Autodesk Inventor part; units mm, degrees
(part 2 of 2)
extrude "Extrusion24" cut sketch "Sketch28" against normal blind 1 contours L33 L34 L10 L12 | L12 L10 S18 L36 L29 L30 L31 L32 L33 | L12 L35 S16 S17 S18 L10 | L10 L34 L35 L12 | S2 S3 S4 S5 L13 L14 S6 S7 S8 S9 L10 | L10 S9 S10 S11 S12 S13 L15 L16 S14 S15 S0 S1 S2 | L26 L27 L28 L17 L18 L19 L20 L10 | L10 L20 L21 L22 L23 L24 L25 L26 | S25 S26 S27 S28 L40 L41 S29 S30 S31 S32 L10 | L10 S32 S33 S34 S35 S36 L42 L43 S37 S38 S23 S24 S25 bodies 3
chamfer "Chamfer2" distance 0.5 angle 45 69 edges at (3.5434, 22.1781, 13.5) (1.331, 22.8406, 13.5) (-2.8323, 22.4212, 13.5) (-6.3513, 18.4524, 13.5) (-6.3391, 11.8155, 13.5) (-2.814, 7.9075, 13.5) (1.3371, 7.5246, 13.5) (3.6102, 8.26, 13.5) (4.5462, 9.8949, 13.5) (3.7622, 10.527, 13.5) (4.4733, 11.0861, 13.5) (3.7075, 19.8625, 13.5) (1.4526, 21.0476, 13.5) (-1.9145, 20.8532, 13.5) (-4.4003, 17.7778, 13.5) (-4.3821, 12.5144, 13.5) (-1.8902, 9.5181, 13.5) (1.5012, 9.354, 13.5) (4.4672, 19.279, 13.5) (4.5462, 20.4824, 13.5) (5.8225, 21.9168, 13.5) (8.7277, 22.6826, 13.5) (6.7767, 21.151, 13.5) (7.731, 15.1826, 13.5) (9.7245, 15.1826, 13.5) (10.6787, 21.151, 13.5) (11.6329, 21.9168, 13.5) (8.7277, 7.6826, 13.5) (11.6329, 8.4484, 13.5) (10.6787, 9.2142, 13.5) (6.7767, 9.2142, 13.5) (5.8225, 8.4484, 13.5) (14.1005, 15.1826, 13.5) (16.0332, 22.6826, 13.5) (20.1236, 22.5428, 13.5) (23.0288, 20.5857, 13.5) (22.6459, 15.8572, 13.5) (16.9692, 15.3163, 13.5) (19.3942, 15.4682, 13.5) (16.094, 18.1364, 13.5) (19.4672, 20.841, 13.5) (17.0847, 20.9565, 13.5) (21.175, 19.6133, 13.5) (21.1994, 17.091, 13.5) (17.2366, 13.651, 13.5) (20.7496, 10.6668, 13.5) (16.094, 10.6668, 13.5) (15.0972, 7.6826, 13.5) (23.0409, 10.9464, 13.5) (24.4145, 7.6826, 13.5) (26.5417, 11.8155, 13.5) (26.5296, 18.4524, 13.5) (28.4988, 12.5144, 13.5) (28.4806, 17.7778, 13.5) (30.0669, 7.9075, 13.5) (34.218, 7.5246, 13.5) (30.9907, 9.5181, 13.5) (34.3821, 9.354, 13.5) (30.0486, 22.4212, 13.5) (34.2119, 22.8406, 13.5) (30.9664, 20.8532, 13.5) (34.3335, 21.0476, 13.5) (36.5883, 19.8625, 13.5) (37.4271, 20.4824, 13.5) (36.4242, 22.1781, 13.5) (37.4271, 9.8949, 13.5) (36.643, 10.527, 13.5) (36.4911, 8.26, 13.5) (37.3541, 11.0861, 13.5)
sketch "Sketch29" plane through (20, -26.8311, -2) normal (0.5, -0.8660254, 0) x (0.8660254, 0.5, 0)
  line L0 (33.3708, 0) -> (0, 0) projected
  line L1 (0, 7.25) -> (0, 0) projected
  line L2 (0, 7.25) -> (12.2679, 7.25) projected
  arc A0 (12.2679, 7.25) -> (16, 6.25) centre (14, 6.25) ccw projected
  arc A1 (16, 6.25) -> (15.7321, 7.25) centre (14, 6.25) ccw projected
  line L3 (15.7321, 7.25) -> (16.2679, 7.25) projected
  arc A2 (16.2679, 7.25) -> (16, 6.25) centre (18, 6.25) ccw projected
  line L4 (33.3708, 7.25) -> (33.3708, 0) projected
  line L5 (19.7321, 7.25) -> (33.3708, 7.25) projected
  arc A3 (16, 6.25) -> (19.7321, 7.25) centre (18, 6.25) ccw projected
  line L6 (0, 12.5) -> (33.3708, 12.5) projected
  line L7 (33.3708, 7.25) -> (33.3708, 12.5) projected
  line L8 (33.3708, 7.25) -> (19.7321, 7.25) projected
  arc A4 (19.7321, 7.25) -> (16.2679, 7.25) centre (18, 6.25) ccw projected
  line L9 (16.2679, 7.25) -> (15.7321, 7.25) projected
  arc A5 (15.7321, 7.25) -> (12.2679, 7.25) centre (14, 6.25) ccw projected
  line L10 (12.2679, 7.25) -> (0, 7.25) projected
  line L11 (0, 7.25) -> (0, 12.5) projected
  line L12 (16.2679, 5.25) -> (15.7321, 5.25) projected
  arc A6 (17.3708, 6.25) -> (17.6388, 5.25) centre (19.3708, 6.25) ccw projected
  arc A7 (17.1029, 5.25) -> (17.3708, 6.25) centre (15.3708, 6.25) ccw projected
  line L13 (17.1029, 5.25) -> (17.6388, 5.25) projected
  line L14 (13.3708, 10.5) -> (13.3708, 6.25) projected
  arc A8 (17.3708, 6.25) -> (13.3708, 6.25) centre (15.3708, 6.25) ccw projected
  arc A9 (21.1029, 5.25) -> (17.3708, 6.25) centre (19.3708, 6.25) ccw projected
  line L15 (21.1029, 5.25) -> (33.3708, 5.25) projected
  line L16 (33.3708, 5.25) -> (33.3708, 10.5) projected
  line L17 (33.3708, 10.5) -> (13.3708, 10.5) projected
  line L18 (17.6388, 7.25) -> (17.1029, 7.25) projected
  point P0 (-3.905, 2)
  point P1 (17.3708, 6.25)
  point P2 (17.3708, 6.25)
  point P3 (17.3708, 6.25)
  point P4 (17.3708, 6.25)
extrude "Extrusion25" cut sketch "Sketch29" along normal through all both and the other way through all contours A0 A3 L12 | A6 L13 A7 | A1 L3 A2 | A9 A8 L18 bodies 3 2
sketch "Sketch30" plane through (-18.9, -10.1457, -2) normal (-0.5, -0.8660254, 0) x (0.8660254, -0.5, 0)
  arc A0 (17.6388, 7.25) -> (17.3708, 6.25) centre (19.3708, 6.25) ccw projected
  arc A1 (17.3708, 6.25) -> (17.1029, 7.25) centre (15.3708, 6.25) ccw projected
  line L0 (17.1029, 7.25) -> (17.6388, 7.25) projected
  arc A2 (17.3708, 6.25) -> (21.1029, 7.25) centre (19.3708, 6.25) ccw projected
  line L1 (21.1029, 7.25) -> (33.3708, 7.25) projected
  line L2 (33.3708, 7.25) -> (33.3708, 0) projected
  line L3 (33.3708, 0) -> (0, 0) projected
  line L4 (0, 0) -> (0, 7.25) projected
  line L5 (0, 7.25) -> (13.6388, 7.25) projected
  arc A3 (13.6388, 7.25) -> (17.3708, 6.25) centre (15.3708, 6.25) ccw projected
  line L6 (0, 12.5) -> (33.3708, 12.5) projected
  line L7 (33.3708, 7.25) -> (33.3708, 12.5) projected
  line L8 (33.3708, 7.25) -> (21.1029, 7.25) projected
  arc A4 (21.1029, 7.25) -> (17.6388, 7.25) centre (19.3708, 6.25) ccw projected
  line L9 (17.6388, 7.25) -> (17.1029, 7.25) projected
  arc A5 (17.1029, 7.25) -> (13.6388, 7.25) centre (15.3708, 6.25) ccw projected
  line L10 (13.6388, 7.25) -> (0, 7.25) projected
  line L11 (0, 7.25) -> (0, 12.5) projected
  arc A6 (15.7321, 5.25) -> (16, 6.25) centre (14, 6.25) ccw projected
  line L12 (15.7321, 5.25) -> (16.2679, 5.25) projected
  arc A7 (16, 6.25) -> (16.2679, 5.25) centre (18, 6.25) ccw projected
  line L13 (16.2679, 7.25) -> (15.7321, 7.25) projected
  line L14 (17.6388, 5.25) -> (17.1029, 5.25) projected
  line L15 (20, 6.25) -> (20, 10.5) projected
  line L16 (20, 10.5) -> (0, 10.5) projected
  line L17 (0, 5.25) -> (0, 10.5) projected
  line L18 (0, 5.25) -> (12.2679, 5.25) projected
  arc A8 (16, 6.25) -> (12.2679, 5.25) centre (14, 6.25) ccw projected
  arc A9 (20, 6.25) -> (16, 6.25) centre (18, 6.25) ccw projected
  point P0 (11.295, 2)
  point P1 (16, 6.25)
  point P2 (16, 6.25)
  point P3 (16, 6.25)
  point P4 (16, 6.25)
  point P5 (16.2679, 7.25)
extrude "Extrusion26" cut sketch "Sketch30" along normal through all both and the other way through all contours A0 A1 L0 | A7 L12 A6 | A2 L14 A3 | A9 A8 L13 bodies 3 2
sketch "Sketch31" plane through (14.1005, 22.6826, 12.5) normal (0, -1, 0) x (1, 0, 0)
  spline S0 degree 6 poles (0.6316, -7.25) (0.7223, -7.4071) (0.7938, -7.5704) (0.8468, -7.7378) (0.8819, -7.9077) (0.8995, -8.0788) (0.8995, -8.25) knots 0 0 0 0 0 0 0 1 1 1 1 1 1 1 projected
  spline S1 degree 6 poles (0.8995, -8.25) (0.8995, -8.0788) (0.9171, -7.9077) (0.9522, -7.7378) (1.0053, -7.5704) (1.0768, -7.4071) (1.1675, -7.25) knots 0 0 0 0 0 0 0 1 1 1 1 1 1 1 projected
  line L0 (0.6316, -7.25) -> (1.1675, -7.25) projected
  line L1 (5.8995, -14.5) -> (-4.1005, -14.5) projected
  line L2 (5.8995, -14.5) -> (5.8995, -7.25) projected
  line L3 (4.6316, -7.25) -> (5.8995, -7.25) projected
  spline S2 degree 8 poles (4.6316, -7.25) (4.8369, -7.6063) (4.9535, -7.9979) (4.9767, -8.4107) (4.9123, -8.811) (4.7612, -9.2007) (4.5177, -9.5581) (4.1783, -9.8586) (3.5089, -10.1736) (3.2342, -10.2576) (2.9375, -10.2969) (2.633, -10.2838) (2.3363, -10.2177) (2.0625, -10.104) (1.8232, -9.9553) (1.4376, -9.6363) (1.2799, -9.4621) (1.1509, -9.2744) (1.0494, -9.0775) (0.9742, -8.8743) (0.9244, -8.6675) (0.8995, -8.4588) (0.8995, -8.25) knots 0 0 0 0 0 0 0 0 0 0.475976 0.475976 0.475976 0.475976 0.475976 0.475976 0.475976 0.745775 0.745775 0.745775 0.745775 0.745775 0.745775 0.745775 1 1 1 1 1 1 1 1 1 projected
  spline S3 degree 7 poles (0.8995, -8.25) (0.8995, -8.4654) (0.8725, -8.6809) (0.8183, -8.8922) (0.7378, -9.0954) (0.6327, -9.2865) (0.5049, -9.462) (0.21, -9.7761) (0.0428, -9.9147) (-0.1414, -10.0317) (-0.3391, -10.1247) (-0.5466, -10.192) (-0.7599, -10.2325) (-1.2499, -10.2634) (-1.5194, -10.2359) (-1.7754, -10.1681) (-2.0114, -10.0653) (-2.2224, -9.9341) (-2.405, -9.7825) (-2.7157, -9.4516) (-2.8461, -9.2677) (-2.9497, -9.072) (-3.0267, -8.868) (-3.0775, -8.6586) (-3.1021, -8.4465) (-3.0996, -8.1251) (-3.0918, -8.016) (-3.077, -7.9073) (-3.0553, -7.7994) (-3.0266, -7.6927) (-2.9909, -7.5877) (-2.934, -7.4504) (-2.9191, -7.4163) (-2.9033, -7.3825) (-2.8868, -7.3489) (-2.8695, -7.3157) (-2.8514, -7.2827) (-2.8325, -7.25) knots 0 0 0 0 0 0 0 0 0.182267 0.182267 0.182267 0.182267 0.182267 0.182267 0.364458 0.364458 0.364458 0.364458 0.364458 0.364458 0.597395 0.597395 0.597395 0.597395 0.597395 0.597395 0.836244 0.836244 0.836244 0.836244 0.836244 0.836244 0.959121 0.959121 0.959121 0.959121 0.959121 0.959121 1 1 1 1 1 1 1 1 projected
  line L4 (-4.1005, -7.25) -> (-2.8325, -7.25) projected
  line L5 (-4.1005, -14.5) -> (-4.1005, -7.25) projected
  line L6 (0.6316, -9.25) -> (1.1675, -9.25) projected
  point P0 (-14.1005, -12.5)
  constraints: 4 other
extrude "Extrusion27" cut sketch "Sketch31" along normal blind 100 contours L0 S1 S0 | S2 L6 S3 bodies 3 2
ref_plane "Work Plane8" through (15, 0, 0) normal (1, 0, 0) x (0, 0, -1)
ref_plane "Work Plane11" through (15, 30.4, 0) normal (-1, 0, 0) x (0, 0, -1)
ref_plane "Work Plane12" through (15, 30.4, 0) normal (-1, 0, 0) x (0, 0, -1)
equation "\"d4\" = d0"
body "Solid1"
